Autodesk Fusion 360 part; units mm, degrees
(part 2 of 2)
  measures "d49" diameter of A26
  measures "d50" diameter of A35
  measures "d51" diameter of A27
  measures "d52" diameter of A32
  measures "d53" diameter of A33
  measures "d54" diameter of A34
  measures "d55" distance of A35.centre A26.centre
  measures "d56" distance of A26.centre A27.centre
  measures "d57" distance of A27.centre A33.centre
  measures "d58" horizontal distance of A22.centre A19.centre
  measures "d59" horizontal distance of A24.centre A26.centre
  measures "d60" distance of A4.centre A18.centre
  measures "d61" diameter of A40
  measures "d62" diameter of A39
  measures "d63" diameter of A41
  measures "d64" diameter of A42
  measures "d65" diameter of A50
  measures "d66" diameter of A52
  measures "d67" distance of A39.centre A40.centre
  measures "d68" distance of A41.centre A40.centre
  measures "d69" distance of A41.centre A50.centre
  measures "d70" diameter of A51
  measures "d71" diameter of A37
  measures "d72" diameter of A38
  measures "d73" diameter of A55
  measures "d74" diameter of A53
  measures "d75" diameter of A58
  measures "d76" distance of A37.centre A51.centre
  measures "d77" distance of A38.centre A51.centre
  measures "d78" distance of A38.centre A53.centre
  measures "d79" diameter of A36
  measures "d80" diameter of A56
  measures "d81" diameter of A43
  measures "d82" diameter of A44
  measures "d83" diameter of A57
  measures "d84" diameter of A60
  measures "d85" distance of A56.centre A36.centre
  measures "d86" distance of A36.centre A43.centre
  measures "d87" distance of A43.centre A57.centre
  measures "d88" horizontal distance of A51.centre A39.centre
  measures "d89" horizontal distance of A37.centre A36.centre
  measures "d90" diameter of A48
  measures "d91" diameter of A49
  measures "d92" diameter of A70
  measures "d93" diameter of A66
  measures "d94" diameter of A71
  measures "d95" diameter of A69
  measures "d96" distance of A48.centre A49.centre
  measures "d97" distance of A48.centre A70.centre
  measures "d98" distance of A71.centre A70.centre
  measures "d99" diameter of A54
  measures "d100" diameter of A59
  measures "d101" diameter of A67
  measures "d102" diameter of A63
  measures "d103" diameter of A68
  measures "d104" diameter of A64
  measures "d105" distance of A59.centre A54.centre
  measures "d106" distance of A67.centre A54.centre
  measures "d107" distance of A67.centre A68.centre
  measures "d108" diameter of A61
  measures "d109" diameter of A45
  measures "d110" diameter of A62
  measures "d111" diameter of A46
  measures "d112" diameter of A65
  measures "d113" diameter of A47
  measures "d114" distance of A45.centre A61.centre
  measures "d115" distance of A61.centre A62.centre
  measures "d116" distance of A62.centre A65.centre
  measures "d117" horizontal distance of A54.centre A49.centre
  measures "d118" horizontal distance of A59.centre A61.centre
  measures "d119" distance of A48.centre A50.centre
  measures "d120" diameter of A87
  measures "d121" diameter of A88
  measures "d122" diameter of A86
  measures "d123" diameter of A94
  measures "d124" diameter of A85
  measures "d125" diameter of A95
  measures "d126" distance of A88.centre A87.centre
  measures "d127" distance of A86.centre A87.centre
  measures "d128" distance of A86.centre A85.centre
  measures "d129" diameter of A89
  measures "d130" diameter of A90
  measures "d131" diameter of A92
  measures "d132" diameter of A91
  measures "d133" diameter of A93
  measures "d134" diameter of A96
  measures "d135" distance of A90.centre A89.centre
  measures "d136" distance of A92.centre A89.centre
  measures "d137" distance of A92.centre A93.centre
  measures "d138" diameter of A73
  measures "d139" diameter of A72
  measures "d140" diameter of A74
  measures "d141" diameter of A97
  measures "d142" diameter of A75
  measures "d143" diameter of A98
  measures "d144" distance of A72.centre A73.centre
  measures "d145" distance of A73.centre A74.centre
  measures "d146" distance of A74.centre A75.centre
  measures "d147" horizontal distance of A88.centre A89.centre
  measures "d148" horizontal distance of A90.centre A73.centre
  measures "d149" diameter of A84
  measures "d150" diameter of A83
  measures "d151" diameter of A82
  measures "d152" diameter of A107
  measures "d153" diameter of A81
  measures "d154" diameter of A80
  measures "d155" distance of A83.centre A84.centre
  measures "d156" distance of A82.centre A84.centre
  measures "d157" distance of A81.centre A82.centre
  measures "d158" diameter of A106
  measures "d159" diameter of A104
  measures "d160" diameter of A105
  measures "d161" diameter of A103
  measures "d162" diameter of A79
  measures "d163" diameter of A102
  measures "d164" distance of A104.centre A106.centre
  measures "d165" distance of A106.centre A105.centre
  measures "d166" distance of A79.centre A105.centre
  measures "d167" diameter of A76
  measures "d168" diameter of A99
  measures "d169" diameter of A77
  measures "d170" diameter of A100
  measures "d171" diameter of A78
  measures "d172" diameter of A101
  measures "d173" distance of A99.centre A76.centre
  measures "d174" distance of A76.centre A77.centre
  measures "d175" distance of A77.centre A78.centre
  measures "d176" horizontal distance of A106.centre A83.centre
  measures "d177" horizontal distance of A104.centre A76.centre
  measures "d178" distance of A85.centre A84.centre
  measures "d199" diameter of A108
  measures "d200" diameter of A109
  measures "d201" diameter of A111
  measures "d202" diameter of A110
  measures "d203" diameter of A112
  measures "d204" diameter of A113
  measures "d208" horizontal distance of A109.centre A108.centre
  measures "d209" vertical distance of A111.centre A108.centre
  measures "d210" vertical distance of A111.centre A112.centre
  measures "d211" diameter of A114
  measures "d212" diameter of A119
  measures "d213" diameter of A118
  measures "d214" diameter of A115
  measures "d215" diameter of A117
  measures "d216" diameter of A116
  measures "d217" horizontal distance of A114.centre A119.centre
  measures "d218" vertical distance of A114.centre A118.centre
  measures "d219" vertical distance of A118.centre A117.centre
  measures "d220" diameter of A120
  measures "d221" diameter of A125
  measures "d222" diameter of A121
  measures "d223" diameter of A124
  measures "d224" diameter of A122
  measures "d225" diameter of A123
  measures "d226" horizontal distance of A125.centre A120.centre
  measures "d227" vertical distance of A120.centre A121.centre
  measures "d228" vertical distance of A122.centre A121.centre
  measures "d229" distance of A109.centre A114.centre
  measures "d230" horizontal distance of A119.centre A120.centre
  measures "d231" diameter of A126
  measures "d232" diameter of A127
  measures "d233" diameter of A132
  measures "d234" diameter of A130
  measures "d235" diameter of A133
  measures "d236" diameter of A129
  measures "d237" horizontal distance of A126.centre A127.centre
  measures "d238" vertical distance of A126.centre A132.centre
  measures "d239" vertical distance of A132.centre A133.centre
  measures "d240" diameter of A131
  measures "d241" diameter of A134
  measures "d242" diameter of A128
  measures "d243" diameter of A135
  measures "d244" diameter of A136
  measures "d245" diameter of A137
  measures "d246" horizontal distance of A134.centre A131.centre
  measures "d247" vertical distance of A131.centre A128.centre
  measures "d248" vertical distance of A136.centre A128.centre
  measures "d249" diameter of A138
  measures "d250" diameter of A139
  measures "d251" diameter of A140
  measures "d252" diameter of A142
  measures "d253" diameter of A141
  measures "d254" diameter of A143
  measures "d255" horizontal distance of A138.centre A139.centre
  measures "d256" vertical distance of A140.centre A138.centre
  measures "d257" vertical distance of A140.centre A141.centre
  measures "d258" distance of A131.centre A127.centre
  measures "d259" horizontal distance of A134.centre A138.centre
  measures "d260" distance of A112.centre A126.centre
  measures "d261" diameter of A144
  measures "d262" diameter of A145
  measures "d263" diameter of A177
  measures "d264" diameter of A147
  measures "d265" diameter of A146
  measures "d266" diameter of A150
  measures "d267" horizontal distance of A144.centre A145.centre
  measures "d268" vertical distance of A144.centre A177.centre
  measures "d269" vertical distance of A177.centre A146.centre
  measures "d270" diameter of A148
  measures "d271" diameter of A179
  measures "d272" diameter of A149
  measures "d273" diameter of A153
  measures "d274" diameter of A154
  measures "d275" diameter of A156
  measures "d276" horizontal distance of A179.centre A148.centre
  measures "d277" vertical distance of A148.centre A149.centre
  measures "d278" vertical distance of A154.centre A149.centre
  measures "d279" diameter of A178
  measures "d280" diameter of A157
  measures "d281" diameter of A158
  measures "d282" diameter of A164
  measures "d283" diameter of A165
  measures "d284" diameter of A169
  measures "d285" horizontal distance of A178.centre A157.centre
  measures "d286" vertical distance of A158.centre A178.centre
  measures "d287" vertical distance of A158.centre A165.centre
  measures "d288" distance of A148.centre A145.centre
  measures "d289" horizontal distance of A179.centre A178.centre
  measures "d290" diameter of A176
  measures "d291" diameter of A152
  measures "d292" diameter of A151
  measures "d293" diameter of A155
  measures "d294" diameter of A175
  measures "d295" diameter of A160
  measures "d296" horizontal distance of A152.centre A176.centre
  measures "d297" vertical distance of A151.centre A176.centre
  measures "d298" vertical distance of A151.centre A175.centre
  measures "d299" diameter of A159
  measures "d300" diameter of A163
  measures "d301" diameter of A173
  measures "d302" diameter of A174
  measures "d303" diameter of A172
  measures "d304" diameter of A167
  measures "d305" horizontal distance of A159.centre A163.centre
  measures "d306" vertical distance of A159.centre A173.centre
  measures "d307" vertical distance of A172.centre A173.centre
  measures "d308" diameter of A166
  measures "d309" diameter of A161
  measures "d310" diameter of A168
  measures "d311" diameter of A170
  measures "d312" diameter of A162
  measures "d313" diameter of A171
  measures "d314" horizontal distance of A166.centre A161.centre
  measures "d315" vertical distance of A168.centre A166.centre
  measures "d316" vertical distance of A168.centre A162.centre
  measures "d317" distance of A152.centre A159.centre
  measures "d318" horizontal distance of A166.centre A163.centre
  measures "d319" distance of A176.centre A146.centre
  measures "d349" diameter of A180
  measures "d350" diameter of A181
  measures "d351" diameter of A197
  measures "d352" diameter of A184
  measures "d353" diameter of A182
  measures "d354" diameter of A183
  measures "d355" horizontal distance of A176.centre A152.centre
  measures "d356" vertical distance of A176.centre A151.centre
  measures "d357" vertical distance of A151.centre A175.centre
  measures "d358" diameter of A196
  measures "d359" diameter of A195
  measures "d360" diameter of A185
  measures "d361" diameter of A190
  measures "d362" diameter of A186
  measures "d363" diameter of A187
  measures "d364" horizontal distance of A159.centre A163.centre
  measures "d365" vertical distance of A159.centre A173.centre
  measures "d366" vertical distance of A172.centre A173.centre
  measures "d367" diameter of A194
  measures "d368" diameter of A188
  measures "d369" diameter of A189
  measures "d370" diameter of A193
  measures "d371" diameter of A191
  measures "d372" diameter of A192
  measures "d373" horizontal distance of A161.centre A166.centre
  measures "d374" vertical distance of A168.centre A166.centre
  measures "d375" vertical distance of A168.centre A162.centre
  measures "d376" distance of A159.centre A152.centre
  measures "d377" horizontal distance of A166.centre A163.centre
  measures "d408" diameter of A215
  measures "d409" diameter of A202
  measures "d410" diameter of A213
  measures "d411" diameter of A220
  measures "d412" diameter of A203
  measures "d413" diameter of A206
  measures "d414" horizontal distance of A214.centre A201.centre
  measures "d415" vertical distance of A214.centre A212.centre
  measures "d416" vertical distance of A212.centre A203.centre
  measures "d417" diameter of A208
  measures "d418" diameter of A240
  measures "d419" diameter of A249
  measures "d420" diameter of A242
  measures "d421" diameter of A246
  measures "d422" diameter of A245
  measures "d423" horizontal distance of A208.centre A240.centre
  measures "d424" vertical distance of A208.centre A248.centre
  measures "d425" vertical distance of A246.centre A248.centre
  measures "d426" diameter of A232
  measures "d427" diameter of A229
  measures "d428" diameter of A233
  measures "d429" diameter of A224
  measures "d430" diameter of A250
  measures "d431" diameter of A223
  measures "d432" horizontal distance of A228.centre A231.centre
  measures "d433" vertical distance of A233.centre A231.centre
  measures "d434" vertical distance of A233.centre A250.centre
  measures "d435" distance of A208.centre A201.centre
  measures "d436" horizontal distance of A231.centre A240.centre
  measures "d438" diameter of A198
  measures "d439" diameter of A216
  measures "d440" diameter of A199
  measures "d441" diameter of A200
  measures "d442" diameter of A217
  measures "d443" diameter of A211
  measures "d444" horizontal distance of A216.centre A198.centre
  measures "d445" vertical distance of A199.centre A198.centre
  measures "d446" vertical distance of A199.centre A217.centre
  measures "d447" diameter of A218
  measures "d448" diameter of A238
  measures "d449" diameter of A239
  measures "d450" diameter of A237
  measures "d451" diameter of A210
  measures "d452" diameter of A207
  measures "d453" horizontal distance of A238.centre A218.centre
  measures "d454" vertical distance of A218.centre A239.centre
  measures "d455" vertical distance of A239.centre A210.centre
  measures "d456" diameter of A236
  measures "d457" diameter of A226
  measures "d458" diameter of A235
  measures "d459" diameter of A230
  measures "d460" diameter of A221
  measures "d461" diameter of A227
  measures "d462" horizontal distance of A236.centre A226.centre
  measures "d463" vertical distance of A235.centre A236.centre
  measures "d464" vertical distance of A235.centre A221.centre
  measures "d465" distance of A216.centre A218.centre
  measures "d466" horizontal distance of A236.centre A238.centre
  measures "d467" diameter of A214
  measures "d468" diameter of A201
  measures "d469" diameter of A212
  measures "d470" diameter of A219
  measures "d471" diameter of A204
  measures "d472" diameter of A205
  measures "d473" horizontal distance of A214.centre A201.centre
  measures "d474" vertical distance of A214.centre A212.centre
  measures "d475" vertical distance of A212.centre A203.centre
  measures "d476" diameter of A209
  measures "d477" diameter of A241
  measures "d478" diameter of A248
  measures "d479" diameter of A243
  measures "d480" diameter of A247
  measures "d481" diameter of A244
  measures "d482" horizontal distance of A208.centre A240.centre
  measures "d483" vertical distance of A208.centre A248.centre
  measures "d484" vertical distance of A246.centre A248.centre
  measures "d485" diameter of A231
  measures "d486" diameter of A228
  measures "d487" diameter of A234
  measures "d488" diameter of A225
  measures "d489" diameter of A251
  measures "d490" diameter of A222
  measures "d491" horizontal distance of A228.centre A231.centre
  measures "d492" vertical distance of A233.centre A231.centre
  measures "d493" vertical distance of A233.centre A250.centre
  measures "d494" distance of A208.centre A201.centre
  measures "d495" horizontal distance of A231.centre A240.centre
  measures "d496" distance of A214.centre A217.centre
  measures "d503" diameter of A305
  measures "d504" diameter of A287
  measures "d505" diameter of A301
  measures "d506" diameter of A263
  measures "d507" diameter of A302
  measures "d508" diameter of A268
  measures "d509" horizontal distance of A304.centre A258.centre
  measures "d510" vertical distance of A304.centre A301.centre
  measures "d511" vertical distance of A301.centre A300.centre
  measures "d512" diameter of A286
  measures "d513" diameter of A255
  measures "d514" diameter of A266
  measures "d515" diameter of A295
  measures "d516" diameter of A265
  measures "d517" diameter of A292
  measures "d518" horizontal distance of A255.centre A259.centre
  measures "d519" vertical distance of A266.centre A259.centre
  measures "d520" vertical distance of A260.centre A266.centre
  measures "d521" diameter of A253
  measures "d522" diameter of A269
  measures "d523" diameter of A290
  measures "d524" diameter of A261
  measures "d525" diameter of A257
  measures "d526" diameter of A270
  measures "d527" horizontal distance of A253.centre A252.centre
  measures "d528" vertical distance of A253.centre A254.centre
  measures "d529" vertical distance of A257.centre A254.centre
  measures "d530" distance of A258.centre A259.centre
  measures "d531" horizontal distance of A253.centre A255.centre
  measures "d532" diameter of A297
  measures "d533" diameter of A280
  measures "d534" diameter of A298
  measures "d535" diameter of A281
  measures "d536" diameter of A299
  measures "d537" diameter of A275
  measures "d538" horizontal distance of A297.centre A280.centre
  measures "d539" vertical distance of A298.centre A297.centre
  measures "d540" vertical distance of A298.centre A299.centre
  measures "d541" diameter of A277
  measures "d542" diameter of A283
  measures "d543" diameter of A273
  measures "d544" diameter of A279
  measures "d545" diameter of A274
  measures "d546" diameter of A282
  measures "d547" horizontal distance of A283.centre A277.centre
  measures "d548" vertical distance of A273.centre A277.centre
  measures "d549" vertical distance of A273.centre A274.centre
  measures "d550" diameter of A272
  measures "d551" diameter of A271
  measures "d552" diameter of A285
  measures "d553" diameter of A284
  measures "d554" diameter of A276
  measures "d555" diameter of A278
  measures "d556" horizontal distance of A272.centre A271.centre
  measures "d557" vertical distance of A285.centre A272.centre
  measures "d558" vertical distance of A285.centre A276.centre
  measures "d559" distance of A280.centre A277.centre
  measures "d560" horizontal distance of A272.centre A283.centre
  measures "d561" diameter of A304
  measures "d562" diameter of A258
  measures "d563" diameter of A303
  measures "d564" diameter of A293
  measures "d565" diameter of A300
  measures "d566" diameter of A288
  measures "d567" horizontal distance of A258.centre A304.centre
  measures "d568" vertical distance of A301.centre A304.centre
  measures "d569" vertical distance of A301.centre A300.centre
  measures "d570" diameter of A259
  measures "d571" diameter of A294
  measures "d572" diameter of A296
  measures "d573" diameter of A256
  measures "d574" diameter of A260
  measures "d575" diameter of A291
  measures "d576" horizontal distance of A259.centre A255.centre
  measures "d577" vertical distance of A259.centre A266.centre
  measures "d578" vertical distance of A266.centre A260.centre
  measures "d579" diameter of A264
  measures "d580" diameter of A252
  measures "d581" diameter of A254
  measures "d582" diameter of A262
  measures "d583" diameter of A267
  measures "d584" diameter of A289
  measures "d585" horizontal distance of A252.centre A253.centre
  measures "d586" vertical distance of A254.centre A253.centre
  measures "d587" vertical distance of A254.centre A257.centre
  measures "d588" distance of A259.centre A258.centre
  measures "d589" horizontal distance of A255.centre A253.centre
  measures "d590" distance of A299.centre A304.centre
  measures "d591" diameter of A328
  measures "d592" diameter of A340
  measures "d593" diameter of A332
  measures "d594" diameter of A306
  measures "d595" diameter of A329
  measures "d596" diameter of A308
  measures "d597" distance of A340.centre A328.centre
  measures "d598" distance of A328.centre A332.centre
  measures "d599" distance of A329.centre A332.centre
  measures "d600" diameter of A315
  measures "d601" diameter of A341
  measures "d602" diameter of A338
  measures "d603" diameter of A319
  measures "d604" diameter of A323
  measures "d605" diameter of A335
  measures "d606" distance of A341.centre A315.centre
  measures "d607" distance of A338.centre A315.centre
  measures "d608" distance of A338.centre A323.centre
  measures "d609" diameter of A312
  measures "d610" diameter of A307
  measures "d611" diameter of A309
  measures "d612" diameter of A318
  measures "d613" diameter of A325
  measures "d614" diameter of A330
  measures "d615" distance of A307.centre A312.centre
  measures "d616" distance of A312.centre A309.centre
  measures "d617" distance of A309.centre A325.centre
  measures "d618" horizontal distance of A340.centre A315.centre
  measures "d619" horizontal distance of A341.centre A312.centre
  measures "d620" diameter of A331
  measures "d621" diameter of A314
  measures "d622" diameter of A334
  measures "d623" diameter of A337
  measures "d624" diameter of A313
  measures "d625" diameter of A322
  measures "d626" distance of A331.centre A314.centre
  measures "d627" distance of A334.centre A331.centre
  measures "d628" distance of A334.centre A313.centre
  measures "d629" diameter of A320
  measures "d630" diameter of A336
  measures "d631" diameter of A324
  measures "d632" diameter of A339
  measures "d633" diameter of A317
  measures "d634" diameter of A321
  measures "d635" distance of A336.centre A320.centre
  measures "d636" distance of A324.centre A320.centre
  measures "d637" distance of A324.centre A317.centre
  measures "d638" diameter of A333
  measures "d639" diameter of A310
  measures "d640" diameter of A327
  measures "d641" diameter of A326
  measures "d642" diameter of A316
  measures "d643" diameter of A311
  measures "d644" distance of A333.centre A310.centre
  measures "d645" distance of A333.centre A327.centre
  measures "d646" distance of A327.centre A316.centre
  measures "d647" horizontal distance of A320.centre A314.centre
  measures "d648" horizontal distance of A333.centre A336.centre
  measures "d649" distance of A329.centre A331.centre
extrude "Extrude9" add sketch "Sketch1" along normal blind 0.9 contours A0 | A1 | A2 | A4 | A6 | A7 | A12 | A13 | A14 | A17 | A18 | A23 | A25 | A28 | A30 | A31 | A32 | A33 | A34 | A35 | A40 | A42 | A43 | A47 | A53 | A54 | A56 | A58 | A59 | A62 | A66 | A71 | A75 | A76 | A78 | A79 | A80 | A81 | A82 | A83 | A89 | A90 | A91 | A92 | A95 | A100 | A101 | A102 | A108 | A109 | A111 | A112 | A114 | A119 | A120 | A123 | A124 | A125 | A126 | A129 | A132 | A133 | A136 | A137 | A139 | A141 | A142 | A143 | A144 | A147 | A154 | A155 A184 | A156 | A157 | A158 | A159 A196 | A163 A195 | A168 A189 | A171 A192 | A175 A182 | A201 A202 | A203 A204 | A205 A206 | A211 | A212 A213 | A218 | A221 | A222 A223 | A224 A225 | A231 A232 | A237 | A238 | A239 | A244 A245 | A246 A247 | A250 A251 | A252 A269 | A254 A290 | A260 A265 | A263 A293 | A277 | A278 | A281 | A283 | A285 | A291 A292 | A299 | A304 A305 | A306 | A309 | A310 | A315 | A317 | A321 | A327 | A329 | A330 | A331 | A337 | A341 makes body 1 at (73.0431, -18.8104, 0.6) makes body 2 at (62.9377, -21.2721, 0.6) makes body 3 at (68.0431, -11.3104, 0.6) makes body 4 at (66.2085, 2.9792, 0.6) makes body 5 at (57.4463, 0.0253, 0.3) makes body 6 at (61.7963, 9.8579, 0.6) makes body 7 at (53.9377, -21.2721, 0.6) makes body 8 at (46.4377, -23.7721, 0.6) makes body 9 at (43.9377, -18.7721, 0.6) makes body 10 at (49.2309, -11.4317, 0.6) makes body 11 at (44.0463, -2.3747, 0.3) makes body 12 at (46.3463, 2.2253, 0.3) makes body 13 at (39.4463, 2.3209, 0.3) makes body 14 at (43.7963, 9.8579, 0.6) makes body 15 at (26.4377, -18.7721, 0.6) makes body 16 at (33.9377, -23.7721, 0.6) makes body 17 at (23.9377, -13.7721, 0.6) makes body 18 at (24.2031, 3.022, 0.6) makes body 19 at (31.1031, -1.578, 0.6) makes body 20 at (21.9031, 7.722, 0.6) makes body 21 at (9.9883, -12.5687, 0.6) makes body 22 at (15.9377, -18.216, 0.3) makes body 23 at (7.5759, -24.6354, 0.6) makes body 24 at (3.8746, -24.603, 0.6) makes body 25 at (2.4883, -15.0687, 0.6) makes body 26 at (9.5537, 9.2209, 0.6) makes body 27 at (15.6463, 4.6253, 0.3) makes body 28 at (13.3463, -2.3747, 0.3) makes body 29 at (4.1463, -2.2747, 0.3) makes body 30 at (4.1463, 6.9253, 0.3) makes body 31 at (4.1463, 4.6253, 0.3) makes body 32 at (6.4463, -2.2747, 0.3) makes body 33 at (15.6463, -2.3747, 0.3) makes body 34 at (15.6463, 6.9253, 0.3) makes body 35 at (7.2537, 9.2253, 0.6) makes body 36 at (3.8746, -17.103, 0.6) makes body 37 at (15.9377, -25.716, 0.3) makes body 38 at (6.3746, -24.603, 0.6) makes body 39 at (15.9377, -15.716, 0.3) makes body 40 at (7.4883, -12.5687, 0.6) makes body 41 at (24.2031, 5.422, 0.6) makes body 42 at (31.1031, 10.0175, 0.6) makes body 43 at (21.9031, 0.822, 0.6) makes body 44 at (26.4377, -16.2721, 0.6) makes body 45 at (34.2309, -11.4317, 0.6) makes body 46 at (23.9377, -21.2721, 0.6) makes body 47 at (41.2031, 7.722, 0.6) makes body 48 at (37.1463, 0.0253, 0.3) makes body 49 at (48.6463, -0.0747, 0.3) makes body 50 at (41.7463, -2.3747, 0.3) makes body 51 at (49.2309, -13.9317, 0.6) makes body 52 at (41.4377, -21.2721, 0.6) makes body 53 at (48.9377, -23.7721, 0.6) makes body 54 at (51.4377, -18.7721, 0.6) makes body 55 at (56.9031, 7.722, 0.6) makes body 56 at (59.7463, -2.3747, 0.3) makes body 57 at (66.2085, 5.3836, 0.6) makes body 58 at (63.2309, -13.9317, 0.6) makes body 59 at (65.5431, -23.8104, 0.6) makes body 60 at (73.0431, -16.3104, 0.6) makes body 61 at (70.5431, -21.3104, 0.6) makes body 62 at (60.4377, -18.7721, 0.6) makes body 63 at (65.5431, -11.3104, 0.6) makes body 64 at (64.1745, 0.4821, 0.6) makes body 65 at (55.1463, 2.3253, 0.3) makes body 66 at (59.4963, 9.8623, 0.6) makes body 67 at (53.9377, -23.7721, 0.6) makes body 68 at (43.9377, -23.7721, 0.6) makes body 69 at (43.9377, -16.2721, 0.6) makes body 70 at (46.7309, -11.4317, 0.6) makes body 71 at (46.3463, -2.3747, 0.3) makes body 72 at (45.8031, 5.422, 0.6) makes body 73 at (38.9031, 5.422, 0.6) makes body 74 at (41.4963, 9.8623, 0.6) makes body 75 at (28.9377, -16.2721, 0.6) makes body 76 at (31.4377, -21.2721, 0.6) makes body 77 at (21.4377, -11.2721, 0.6) makes body 78 at (26.5031, 5.422, 0.6) makes body 79 at (28.8031, 0.722, 0.6) makes body 80 at (19.6031, 10.022, 0.6) makes body 81 at (12.4883, -12.5687, 0.6) makes body 82 at (15.9377, -20.716, 0.3) makes body 83 at (10.0435, -25.2854, 0.6) makes body 84 at (3.8746, -22.103, 0.6) makes body 85 at (2.4883, -12.5687, 0.6) makes body 86 at (14.1537, 9.2209, 0.6) makes body 87 at (15.6463, 2.2209, 0.3) makes body 88 at (11.0463, -2.3747, 0.3) makes body 89 at (4.1463, 0.0253, 0.3) makes body 90 at (4.1463, 9.2253, 0.3) makes body 91 at (4.1463, 2.3253, 0.3) makes body 92 at (8.7463, -2.3747, 0.3) makes body 93 at (15.6463, -0.0747, 0.3) makes body 94 at (11.8537, 9.2253, 0.6) makes body 95 at (4.9537, 9.2209, 0.6) makes body 96 at (3.8746, -19.603, 0.6) makes body 97 at (12.5435, -25.2854, 0.6) makes body 98 at (15.9377, -23.216, 0.3) makes body 99 at (15.9377, -13.216, 0.3) makes body 100 at (4.9883, -12.5687, 0.6) makes body 101 at (26.5031, 3.0175, 0.6) makes body 102 at (28.8031, 7.722, 0.6) makes body 103 at (19.6031, -1.478, 0.6) makes body 104 at (28.9377, -18.7721, 0.6) makes body 105 at (31.4377, -13.7721, 0.6) makes body 106 at (21.4377, -23.7721, 0.6) makes body 107 at (43.5031, 7.722, 0.6) makes body 108 at (37.1463, -2.2747, 0.3) makes body 109 at (48.6463, -2.3747, 0.3) makes body 110 at (39.4463, -2.2747, 0.3) makes body 111 at (46.7309, -13.9317, 0.6) makes body 112 at (41.4377, -23.7721, 0.6) makes body 113 at (51.4377, -23.7721, 0.6) makes body 114 at (51.4377, -16.2721, 0.6) makes body 115 at (54.6031, 5.422, 0.6) makes body 116 at (62.0463, -2.3747, 0.3) makes body 117 at (64.1745, 7.4821, 0.6) makes body 118 at (60.4377, -16.2721, 0.6) makes body 119 at (68.0431, -23.8104, 0.6) makes body 120 at (70.5431, -13.8104, 0.6)
extrude "Extrude10" add sketch "Sketch1" 120 faces at (53.7902, -24.2503, 0) (12.8624, -25.0915, 0) (60.2902, -19.2503, 0) (3.2159, -19.7779, 0) (3.1207, -12.7843, 0) (51.2902, -19.2503, 0) (72.7902, -19.2503, 0) (3.2159, -22.2779, 0) (62.7902, -21.7503, 0) (16.1205, -25.0788, 0) (70.2902, -21.7503, 0) (65.2902, -24.2503, 0) (10.5909, -12.0283, 0) (33.7902, -24.2503, 0) (46.179, -14.2503, 0) (67.7902, -24.2503, 0) (5.9818, -12.5313, 0) (67.5706, -11.7448, 0) (8.5711, -24.8856, 0) (43.7902, -16.7503, 0) (13.0909, -12.0283, 0) (31.2545, -22.2268, 0) (48.7902, -24.2503, 0) (46.179, -11.7503, 0) (31.4179, -14.324, 0) (48.679, -14.2503, 0) (3.2159, -17.2779, 0) (41.2902, -24.2503, 0) (15.5676, -11.999, 0) (70.0706, -14.2448, 0) (28.7545, -17.2268, 0) (51.2902, -24.2503, 0) (48.679, -11.7503, 0) (15.5676, -14.499, 0) (43.7902, -19.2503, 0) (23.9179, -14.324, 0) (46.2902, -24.2503, 0) (10.3624, -25.0915, 0) (72.7902, -16.7503, 0) (8.4398, -12.8098, 0) (51.2902, -16.7503, 0) (16.1205, -20.0788, 0) (28.7545, -19.7268, 0) (60.2902, -16.7503, 0) (21.4179, -11.824, 0) (53.7902, -21.7503, 0) (23.7545, -22.2268, 0) (3.2159, -24.7779, 0) (43.7902, -24.2503, 0) (26.2545, -19.7268, 0) (65.0706, -11.7448, 0) (41.2902, -21.7503, 0) (26.2545, -17.2268, 0) (3.1207, -15.2843, 0) (62.679, -14.2503, 0) (16.1205, -22.5788, 0) (21.2545, -24.7268, 0) (43.0329, 7.1955, 0) (33.679, -11.7503, 0) (43.2444, 9.5393, 0) (5.3267, -25.1025, 0) (16.1205, -17.5788, 0) (38.3972, 2.602, 0) (38.4329, 4.8955, 0) (45.3329, 4.8955, 0) (56.4329, 7.1955, 0) (15.1252, 2.404, 0) (40.7329, -2.1045, 0) (19.5805, -2.0672, 0) (40.7329, 7.1955, 0) (28.7722, 0.0964, 0) (31.0805, 9.4283, 0) (63.3329, 7.1955, 0) (24.1722, 4.7964, 0) (40.9444, 9.5437, 0) (3.275, 4.9489, 0) (58.7329, -2.1045, 0) (47.6329, -2.1045, 0) (10.1563, 9.7613, 0) (45.3329, -2.1045, 0) (14.8087, 5.2144, 0) (54.1329, 4.8955, 0) (14.7854, 0.5436, 0) (45.2972, 2.5065, 0) (26.4722, 2.3919, 0) (21.8805, 0.2328, 0) (58.9444, 9.5437, 0) (56.9671, 0.2955, 0) (3.5106, -2.0134, 0) (38.4329, -2.3955, 0) (5.8106, -2.0134, 0) (48.1671, 0.1955, 0) (5.9472, 9.2583, 0) (12.8472, 9.2627, 0) (43.0329, -2.1045, 0) (65.5341, 2.4656, 0) (28.7722, 7.0964, 0) (61.2444, 9.5393, 0) (8.2336, 9.1551, 0) (54.0972, 2.6065, 0) (21.5139, 7.1328, 0) (63.3329, -0.1955, 0) (36.1329, -2.3955, 0) (66.2659, 4.87, 0) (26.4722, 4.7964, 0) (14.8087, 7.5144, 0) (36.6671, 0.2955, 0) (61.0329, -2.1045, 0) (12.8472, -2.3373, 0) (23.8139, 2.4328, 0) (7.7528, -2.3373, 0) (15.1472, -2.3373, 0) (3.4396, 2.6028, 0) (15.1472, 9.2583, 0) (19.5805, 9.4328, 0) (30.7139, -2.1672, 0) (3.5559, 0.2955, 0) (10.5472, -2.3373, 0) (3.5833, 9.5446, 0) (3.0822, 6.8592, 0) against normal blind 6 contours A0 | A1 | A2 | A3 | A4 | A5 | A6 | A7 | A8 | A9 | A10 | A11 | A12 | A13 | A14 | A15 | A16 | A17 | A18 | A19 | A20 | A21 | A22 | A23 | A24 | A25 | A26 | A27 | A28 | A29 | A30 | A31 | A32 | A33 | A34 | A35 | L0 L1 L2 L3 | L4 L5 L6 L7 | A36 | A37 | A38 | A39 | A40 | A41 | A42 | A43 | A44 | A45 | A46 | A47 | A48 | A49 | A50 | A51 | A52 | A53 | A54 | A55 | A56 | A57 | A58 | A59 | A60 | A61 | A62 | A63 | A64 | A65 | A66 | A67 | A68 | A69 | A70 | A71 | L8 L9 L10 L11 | A72 | A73 | A74 | A75 | A76 | A77 | A78 | A79 | A80 | A81 | A82 | A83 | A84 | A85 | A86 | A87 | A88 | A89 | A90 | A91 | A92 | A93 | A94 | A95 | A96 | A97 | A98 | A99 | A100 | A101 | A102 | A103 | A104 | A105 | A106 | A107 | A108 | A109 | A110 | A111 | A112 | A113 | A114 | A115 | A116 | A117 | A118 | A119 | A120 | A121 | A122 | A123 | A124 | A125 | A126 | A127 | A128 | A129 | A130 | A131 | A132 | A133 | A134 | A135 | A136 | A137 | A138 | A139 | A140 | A141 | A142 | A143 | L12 L13 L14 L15 | L16 L17 L18 L19 L20 L21 L22 | A144 | A145 | A146 | A147 | A148 | A149 | A150 | A151 A197 | A152 A181 | A153 | A154 | A155 A184 | A156 | A157 | A158 | A159 A196 | A160 A183 | A161 A188 | A162 A191 | A163 A195 | A164 | A165 | A166 A194 | A167 A187 | A168 A189 | A169 | A170 A193 | A171 A192 | A172 A186 | A173 A185 | A174 A190 | A175 A182 | A176 A180 | A177 | A178 | A179 | L23 L24 L25 L26 L27 L28 L29 | A198 | A199 | A200 | A201 A202 | A203 A204 | A205 A206 | A207 | A208 A209 | A210 | A211 | A212 A213 | A214 A215 | A216 | A217 | A218 | A219 A220 | A221 | A222 A223 | A224 A225 | A226 | A227 | A228 A229 | A230 | A231 A232 | A233 A234 | A235 | A236 | A237 | A238 | A239 | A240 A241 | A242 A243 | A244 A245 | A246 A247 | A248 A249 | A250 A251 | A252 A269 | A253 A264 | A254 A290 | A255 A294 | A256 A295 | A257 A267 | A258 A287 | A259 A286 | A260 A265 | A261 A262 | A263 A293 | A266 A296 | A268 A288 | A270 A289 | A271 | A272 | A273 | A274 | A275 | A276 | A277 | A278 | A279 | A280 | A281 | A282 | A283 | A284 | A285 | L30 L31 L32 L33 L34 L35 L36 | A291 A292 | A297 | A298 | A299 | A300 A302 | A301 A303 | A304 A305 | A306 | A307 | A308 | L37 L38 L39 L40 | A309 | A310 | A311 | A312 | A313 | A314 | A315 | A316 | A317 | A318 | A319 | A320 | A321 | A322 | A323 | A324 | A325 | A326 | A327 | A328 | A329 | A330 | A331 | A332 | A333 | A334 | A335 | A336 | A337 | A338 | A339 | A340 | A341 on bodies 1 2 3 4 5 6 7 8 9 10 11 12 13 14 15 16 17 18 19 20 21 22 23 24 25 26 27 28 29 30 31 32 33 34 35 36 37 38 39 40 41 42 43 44 45 46 47 48 49 50 51 52 53 54 55 56 57 58 59 60 61 62 63 64 65 66 67 68 69 70 71 72 73 74 75 76 77 78 79 80 81 82 83 84 85 86 87 88 89 90 91 92 93 94 95 96 97 98 99 100 101 102 103 104 105 106 107 108 109 110 111 112 113 114 115 116 117 118 119 120 bodies 67 1 4 11 15 18 21 26 2 3 5 6 7 8 9 10 12 13 14 16 17 19 20 22 23 24 25 27 28 29 30 31 32 33 34 35 36 37 38 39 40 41 42 43 44 45 46 47 48 49 50 51 52 53 54 55 56 57 58 59 60 61 62 63 64 65 66 68 69 70 71 72 73 74 75 76 77 78 79 80 81 82 83 84 85 86 87 88 89 90 91 92 93 94 95 96 97 98 99 100 101 102 103 104 105 106 107 108 109 110 111 112 113 114 115 116 117 118 119 120
fillet "Fillet6" radius 0.3 120 edges at (64.5354, -12.2653, 0.9) (67.0354, -12.2653, 0.9) (69.5354, -14.7653, 0.9) (72.0354, -17.2653, 0.9) (72.0354, -19.7653, 0.9) (69.5354, -22.2653, 0.9) (67.0354, -24.7653, 0.9) (64.5354, -24.7653, 0.9) (62.0354, -22.2653, 0.9) (59.5354, -19.7653, 0.9) (59.5354, -17.2653, 0.9) (62.0354, -14.7653, 0.9) (58.3008, 9.0288, 0.9) (60.6008, 9.0243, 0.9) (62.9008, 6.7288, 0.9) (65.2008, 4.4288, 0.9) (65.2008, 2.0243, 0.9) (62.9008, -0.2712, 0.9) (60.6008, -2.5712, 0.9) (58.3008, -2.5712, 0.9) (56.0008, -0.1712, 0.9) (53.7008, 2.1288, 0.9) (53.7008, 4.4288, 0.9) (56.0008, 6.7288, 0.9) (40.3008, 9.0288, 0.9) (42.6008, 9.0243, 0.9) (42.6008, 6.7288, 0.9) (40.3008, 6.7288, 0.9) (38.0008, 4.4288, 0.9) (38.0008, 2.1243, 0.9) (35.7008, -0.1712, 0.9) (35.7008, -2.4712, 0.9) (38.0008, -2.4712, 0.9) (40.3008, -2.5712, 0.9) (42.6008, -2.5712, 0.9) (44.9008, -2.5712, 0.9) (47.2008, -2.5712, 0.9) (47.2008, -0.2712, 0.9) (44.9008, 2.0288, 0.9) (44.9008, 4.4288, 0.9) (33.0354, -24.7653, 0.9) (30.5354, -22.2653, 0.9) (28.0354, -19.7653, 0.9) (28.0354, -17.2653, 0.9) (30.5354, -14.7653, 0.9) (33.0354, -12.2653, 0.9) (20.5354, -12.2653, 0.9) (23.0354, -14.7653, 0.9) (25.5354, -17.2653, 0.9) (25.5354, -19.7653, 0.9) (23.0354, -22.2653, 0.9) (20.5354, -24.7653, 0.9) (18.7008, 9.0288, 0.9) (21.0008, 6.7288, 0.9) (23.3008, 4.4288, 0.9) (25.6008, 4.4288, 0.9) (27.9008, 6.7288, 0.9) (30.2008, 9.0243, 0.9) (23.3008, 2.0288, 0.9) (25.6008, 2.0243, 0.9) (21.0008, -0.1712, 0.9) (18.7008, -2.4712, 0.9) (27.9008, -0.2712, 0.9) (30.2008, -2.5712, 0.9) (2.5354, -12.7653, 0.9) (5.0354, -12.7653, 0.9) (7.5354, -12.7653, 0.9) (10.0354, -12.7653, 0.9) (12.5354, -12.7653, 0.9) (15.0354, -12.7653, 0.9) (15.0354, -15.2653, 0.9) (15.0354, -17.7653, 0.9) (15.0354, -20.2653, 0.9) (15.0354, -22.7653, 0.9) (15.0354, -25.2653, 0.9) (12.5354, -25.2653, 0.9) (10.0354, -25.2653, 0.9) (7.5354, -25.2653, 0.9) (5.0354, -25.2653, 0.9) (2.5354, -25.2653, 0.9) (2.5354, -22.7653, 0.9) (2.5354, -20.2653, 0.9) (2.5354, -17.7653, 0.9) (2.5354, -15.2653, 0.9) (2.7008, 9.0288, 0.9) (5.0008, 9.0243, 0.9) (7.3008, 9.0288, 0.9) (9.6008, 9.0243, 0.9) (11.9008, 9.0288, 0.9) (14.2008, 9.0243, 0.9) (14.2008, 6.7288, 0.9) (14.2008, 4.4288, 0.9) (14.2008, 2.0243, 0.9) (14.2008, -0.2712, 0.9) (14.2008, -2.5712, 0.9) (11.9008, -2.5712, 0.9) (9.6008, -2.5712, 0.9) (7.3008, -2.5712, 0.9) (5.0008, -2.4712, 0.9) (2.7008, -2.4712, 0.9) (2.7008, -0.1712, 0.9) (2.7008, 2.1288, 0.9) (2.7008, 4.4288, 0.9) (2.7008, 6.7288, 0.9) (53.0354, -24.7653, 0.9) (53.0354, -22.2653, 0.9) (50.5354, -19.7653, 0.9) (50.5354, -17.2653, 0.9) (48.0354, -14.7653, 0.9) (48.0354, -12.2653, 0.9) (45.5354, -12.2653, 0.9) (45.5354, -14.7653, 0.9) (43.0354, -17.2653, 0.9) (43.0354, -19.7653, 0.9) (40.5354, -22.2653, 0.9) (40.5354, -24.7653, 0.9) (43.0354, -24.7653, 0.9) (45.5354, -24.7653, 0.9) (48.0354, -24.7653, 0.9) (50.5354, -24.7653, 0.9) on bodies 1 4 11 15 18 21 26 67
